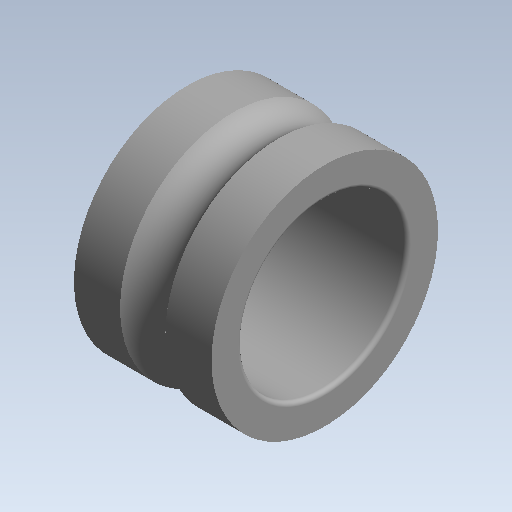
# Autodesk Inventor part: W686ZZ Inner ring
Saved by Autodesk Inventor 2021.3 (Build 253353010, 353A)
## iProperties
Part Number: W686ZZ Inner ring
Material: 一般
Catalog Web Link: www.cadenas.de
Description: Six types ir-Metric system sizes
Vendor: NTN
Document SubType Name: Modeling
Designer: partserver
Manufacturer: NTN
Mass: 0.113494 g
Surface Area: 2.74806 cm^2
Volume: 0.113494 cm^3
Density: 1 g/cm^3
Appearance: PSOLRGB-192-192-192
Category: PARTsolutions
Company: NTN
PSOL_IDENT_0: {$CADENAS_DATA\23d-libs\ntn\ball_roller_bearings\miniature_extra_small_bb\metric_system_sizes\mss_ir
PSOL_IDENT_1: .prj},183 {VTYP=3D},{NB=W686ZZ Inner ring},{LINA=W686ZZ Inner ring},{NN=Six types ir},{DATE=23.10.20
PSOL_IDENT_2: 20 01:13:34},{GEOMDATE=06.03.2020 10:06:06},{VERSION=},{LINEID=12860},{WBVAR=},{WBNUMERIC=}  {NB=W68
PSOL_IDENT_3: 6ZZ Inner ring},{LINA=W686ZZ Inner ring},{KT=DUMMY},{IDNR=},{SD=6.0},{D=13},{B=3.5},{R=0.15},{ORDER=
PSOL_IDENT_4: W686ZZ},{CR=1 080},{COR=440},{CRF=110},{CORF=45},{LSG=39 000},{LSO=46 000},{MASS=1.90},{D1=15.0},{D2=
PSOL_IDENT_5: 15.2},{C1=1.0},{C2=1.1},{ORDER1=686},{WSS=W686ZZ},{WDS=ZZ},{UTWF=FL686},{FORSS=FLW686Z},{FORDS=ZZ},{
PSOL_IDENT_6: DA1=7},{DA2=7,2},{DA=11,8},{RAS=0,15},{MASS1=2.20},{B1=5.0},{VERS=3},{X=3.5},{N=8},{O=29.83},{RB=1.0
PSOL_IDENT_7: 36}
NB: W686ZZ Inner ring
NN: Six types ir
NT: Metric system sizes
NBSYN: $ORDER. Inner ring
LINA: W686ZZ Inner ring
CATALOG: NTN Corporation
SD: 6
D: 13
B: 3.5
R: 0.15
CR: 1 080
COR: 440
CRF: 110
CORF: 45
LSG: 39 000
LSO: 46 000
MASS: 1.9
D1: 15
D2: 15.2
C1: 1
C2: 1.1
ORDER1: 686
WSS: W686ZZ
WDS: ZZ
UTWF: FL686
FORSS: FLW686Z
FORDS: ZZ
DA1: 7
DA2: 7,2
DA: 11,8
RAS: 0,15
MASS1: 2.2
B1: 5
VERS: 3
SUPPLIER: NTN
ARTICLENO: W686ZZ Inner ring
BOMINFO: W686ZZ Inner ring
CREATOR: CADENAS GmbH
Title: W686ZZ Inner ring
Author: Cadenas PARTsolutions
Comments: Metric system sizes
Autodesk Inventor part; units mm, degrees
sketch "Sketch_2" plane through (0, 0, 0) normal (0, 0, 1) x (1, 0, 0)
  line L0 (5, 0) -> (0, 0)
  arc A0 (0, 3.15) -> (0.15, 3) centre (0.15, 3.15) ccw
  line L1 (0.15, 3) -> (4.85, 3)
  arc A1 (4.85, 3) -> (5, 3.15) centre (4.85, 3.15) ccw
  line L2 (5, 3.15) -> (5, 4.12)
  line L3 (5, 4.12) -> (3.3224, 4.12)
  arc A2 (1.6776, 4.12) -> (3.3224, 4.12) centre (2.5, 4.75) ccw
  line L4 (1.6776, 4.12) -> (0, 4.12)
  line L5 (0, 4.12) -> (0, 3.15)
  constraints: 12 end point, 6 point on circle, 3 centre point
revolve "Revolution1" add sketch "Sketch_2" angle 360 about axis through (5, 0, 0) along (1, 0, 0)
ref_plane "mss_ir_XY" through (0, 0, 0) normal (1, 0, 0) x (0, 0, -1)
ref_plane "mss_ir_YZ" through (0, 0, 0) normal (0, 0, -1) x (0, 1, 0)
ref_plane "mss_ir_ZX" through (0, 0, 0) normal (0, 1, 0) x (1, 0, 0)
body "Solid1"
